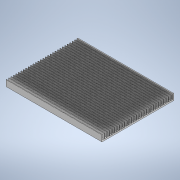
# Autodesk Inventor part: радиатор300х400
Saved by Autodesk Inventor 2020 (Build 240168000, 168)
## iProperties
Created: 2019-11-04
Part Number: радиатор300х400
Material: Типовые
Document SubType Name: Modeling
Designer: Михаил
Density: 1 g/cm^3
Appearance: По умолчанию
Author: Михаил
Autodesk Inventor part; units mm, degrees
ref_plane "YZ Plane" through (0, 0, 0) normal (1, 0, 0) x (0, 1, 0)
ref_plane "XZ Plane" through (0, 0, 0) normal (0, 1, 0) x (-1, 0, 0)
ref_plane "XY Plane" through (0, 0, 0) normal (0, 0, 1) x (1, 0, 0)
sketch "Эскиз1" plane through (0, 0, 0) normal (0, 1, 0) x (-1, 0, 0)
  line L0 (0, 0) -> (400, 0)
  line L1 (400, 0) -> (400, -300)
  line L2 (400, -300) -> (0, -300)
  line L3 (0, -300) -> (0, 0)
  dimension "d0" = 400
  dimension "d1" = 300
  constraints: 8 end point, 2 parallel, 1 horizontal, 1 perpendicular
  measures "d0" distance between parallel lines of L3 L1
  measures "d1" distance between parallel lines of L0 L2
extrude "Выдавливание1" add sketch "Эскиз1" along normal blind 25
sketch "Эскиз2" plane through (0, 0, 0) normal (1, 0, 0) x (0, 0, -1)
  line L0 (0, 25) -> (300, 25) projected
  line L1 (2.2, 25) -> (10.2, 25)
  line L2 (10.2, 25) -> (10.2, 6)
  line L3 (10.2, 6) -> (2.2, 6)
  line L4 (2.2, 6) -> (2.2, 25)
  line L5 (0, 0) -> (0, 25) projected
  line L6 (0, 0) -> (300, 0) projected
  line L7 (20.4, 6) -> (12.4, 6)
  line L8 (20.4, 25) -> (20.4, 6)
  line L9 (12.4, 6) -> (12.4, 25)
  line L10 (12.4, 25) -> (20.4, 25)
  line L11 (30.6, 6) -> (22.6, 6)
  line L12 (30.6, 25) -> (30.6, 6)
  line L13 (22.6, 6) -> (22.6, 25)
  line L14 (22.6, 25) -> (30.6, 25)
  line L15 (40.8, 6) -> (32.8, 6)
  line L16 (40.8, 25) -> (40.8, 6)
  line L17 (32.8, 6) -> (32.8, 25)
  line L18 (32.8, 25) -> (40.8, 25)
  line L19 (51, 6) -> (43, 6)
  line L20 (51, 25) -> (51, 6)
  line L21 (43, 6) -> (43, 25)
  line L22 (43, 25) -> (51, 25)
  line L23 (61.2, 6) -> (53.2, 6)
  line L24 (61.2, 25) -> (61.2, 6)
  line L25 (53.2, 6) -> (53.2, 25)
  line L26 (53.2, 25) -> (61.2, 25)
  line L27 (71.4, 6) -> (63.4, 6)
  line L28 (71.4, 25) -> (71.4, 6)
  line L29 (63.4, 6) -> (63.4, 25)
  line L30 (63.4, 25) -> (71.4, 25)
  line L31 (81.6, 6) -> (73.6, 6)
  line L32 (81.6, 25) -> (81.6, 6)
  line L33 (73.6, 6) -> (73.6, 25)
  line L34 (73.6, 25) -> (81.6, 25)
  line L35 (91.8, 6) -> (83.8, 6)
  line L36 (91.8, 25) -> (91.8, 6)
  line L37 (83.8, 6) -> (83.8, 25)
  line L38 (83.8, 25) -> (91.8, 25)
  line L39 (102, 6) -> (94, 6)
  line L40 (102, 25) -> (102, 6)
  line L41 (94, 6) -> (94, 25)
  line L42 (94, 25) -> (102, 25)
  line L43 (112.2, 6) -> (104.2, 6)
  line L44 (112.2, 25) -> (112.2, 6)
  line L45 (104.2, 6) -> (104.2, 25)
  line L46 (104.2, 25) -> (112.2, 25)
  line L47 (122.4, 6) -> (114.4, 6)
  line L48 (122.4, 25) -> (122.4, 6)
  line L49 (114.4, 6) -> (114.4, 25)
  line L50 (114.4, 25) -> (122.4, 25)
  line L51 (132.6, 6) -> (124.6, 6)
  line L52 (132.6, 25) -> (132.6, 6)
  line L53 (124.6, 6) -> (124.6, 25)
  line L54 (124.6, 25) -> (132.6, 25)
  line L55 (142.8, 6) -> (134.8, 6)
  line L56 (142.8, 25) -> (142.8, 6)
  line L57 (134.8, 6) -> (134.8, 25)
  line L58 (134.8, 25) -> (142.8, 25)
  line L59 (153, 6) -> (145, 6)
  line L60 (153, 25) -> (153, 6)
  line L61 (145, 6) -> (145, 25)
  line L62 (145, 25) -> (153, 25)
  line L63 (163.2, 6) -> (155.2, 6)
  line L64 (163.2, 25) -> (163.2, 6)
  line L65 (155.2, 6) -> (155.2, 25)
  line L66 (155.2, 25) -> (163.2, 25)
  line L67 (173.4, 6) -> (165.4, 6)
  line L68 (173.4, 25) -> (173.4, 6)
  line L69 (165.4, 6) -> (165.4, 25)
  line L70 (165.4, 25) -> (173.4, 25)
  line L71 (183.6, 6) -> (175.6, 6)
  line L72 (183.6, 25) -> (183.6, 6)
  line L73 (175.6, 6) -> (175.6, 25)
  line L74 (175.6, 25) -> (183.6, 25)
  line L75 (193.8, 6) -> (185.8, 6)
  line L76 (193.8, 25) -> (193.8, 6)
  line L77 (185.8, 6) -> (185.8, 25)
  line L78 (185.8, 25) -> (193.8, 25)
  line L79 (204, 6) -> (196, 6)
  line L80 (204, 25) -> (204, 6)
  line L81 (196, 6) -> (196, 25)
  line L82 (196, 25) -> (204, 25)
  line L83 (214.2, 6) -> (206.2, 6)
  line L84 (214.2, 25) -> (214.2, 6)
  line L85 (206.2, 6) -> (206.2, 25)
  line L86 (206.2, 25) -> (214.2, 25)
  line L87 (224.4, 6) -> (216.4, 6)
  line L88 (224.4, 25) -> (224.4, 6)
  line L89 (216.4, 6) -> (216.4, 25)
  line L90 (216.4, 25) -> (224.4, 25)
  line L91 (234.6, 6) -> (226.6, 6)
  line L92 (234.6, 25) -> (234.6, 6)
  line L93 (226.6, 6) -> (226.6, 25)
  line L94 (226.6, 25) -> (234.6, 25)
  line L95 (244.8, 6) -> (236.8, 6)
  line L96 (244.8, 25) -> (244.8, 6)
  line L97 (236.8, 6) -> (236.8, 25)
  line L98 (236.8, 25) -> (244.8, 25)
  line L99 (255, 6) -> (247, 6)
  line L100 (255, 25) -> (255, 6)
  line L101 (247, 6) -> (247, 25)
  line L102 (247, 25) -> (255, 25)
  line L103 (265.2, 6) -> (257.2, 6)
  line L104 (265.2, 25) -> (265.2, 6)
  line L105 (257.2, 6) -> (257.2, 25)
  line L106 (257.2, 25) -> (265.2, 25)
  line L107 (275.4, 6) -> (267.4, 6)
  line L108 (275.4, 25) -> (275.4, 6)
  line L109 (267.4, 6) -> (267.4, 25)
  line L110 (267.4, 25) -> (275.4, 25)
  line L111 (285.6, 6) -> (277.6, 6)
  line L112 (285.6, 25) -> (285.6, 6)
  line L113 (277.6, 6) -> (277.6, 25)
  line L114 (277.6, 25) -> (285.6, 25)
  line L115 (295.8, 6) -> (287.8, 6)
  line L116 (295.8, 25) -> (295.8, 6)
  line L117 (287.8, 6) -> (287.8, 25)
  line L118 (287.8, 25) -> (295.8, 25)
  point P0 (287.8, 25)
  point P1 (277.6, 25)
  point P2 (234.6, 25)
  point P3 (226.6, 25)
  point P4 (185.8, 25)
  point P5 (155.2, 25)
  point P6 (122.4, 25)
  point P7 (102, 25)
  point P8 (73.6, 25)
  point P9 (71.4, 25)
  point P10 (61.2, 25)
  point P11 (30.6, 25)
  dimension "d4" = 2.2
  dimension "d5" = 6
  dimension "d6" = 8
  dimension "d10" = 10.2
  constraints: 232 end point, 2 horizontal, 2 parallel, 1 collinear, 1 perpendicular, 225 other
  measures "d4" distance between parallel lines of L4 L5
  measures "d5" distance between parallel lines of L6 L3
  measures "d6" distance between parallel lines of L4 L2
  measures "d10" distance of L2.end L7.start
extrude "Выдавливание2" cut sketch "Эскиз2" against normal through all
